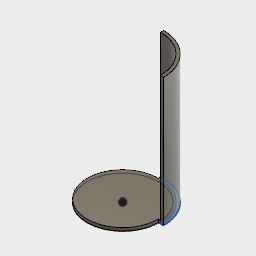
Gelatin_Mold_Remover v1 (Autodesk Fusion 360 design; units mm, degrees)
Autodesk Fusion 360 part; units mm, degrees
sketch "Sketch1" plane through (0, 0, 0) normal (0, 1, 0) x (1, 0, 0)
  circle A0 centre (0, 0) radius 34
  line L0 (0.0039, 39) -> (0.0039, 34)
  line L1 (39, 0.0006) -> (34, 0.0006)
  arc A1 (39, 0.0006) -> (0.0039, 39) centre (0, 0) ccw
  arc A2 (36, 0.0006) -> (0.0039, 36) centre (0, 0) ccw
  dimension "d1" = 68
  measures "d1" diameter of A0
extrude "Extrude1" add sketch "Sketch1" along normal blind 3 contours A0
extrude "Extrude2" add sketch "Sketch1" along normal blind 3 contours A0 L0 L1 A2
extrude "Extrude3" add sketch "Sketch1" along normal blind 123 contours L0 L1 A1 A2
